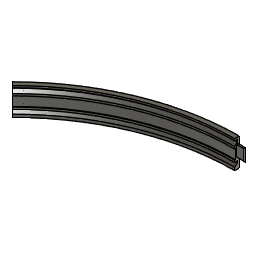
Model_Segment (Autodesk Fusion 360 design; units mm, degrees)
Autodesk Fusion 360 part; units mm, degrees
sketch "Sketch1" plane through (0, 0, 0) normal (0, 0, 1) x (1, 0, 0)
  circle A0 centre (0, 0) radius 246.5
  circle A1 centre (0, 0) radius 241.5
  line L0 (0, 350) -> (0, -350)
  line L1 (-247.4874, 247.4874) -> (247.4874, -247.4874)
  line L2 (-350, 0) -> (350, 0)
  line L3 (-247.4874, -247.4874) -> (247.4874, 247.4874)
  line L4 (0, 350) -> (0, -350)
  circle A2 centre (0, 0) radius 245
  dimension "d2" = 5
  dimension "d3" = 350
  dimension "d4" = 350
  dimension "d5" = 45
  dimension "d6" = 45
  dimension "d7" = 45
  dimension "d8" = 45
  dimension "d50" = 483
  dimension "d64" = 490
  constraint coincident A0.centre A1.centre
  constraint concentric A0 A1
  constraint vertical L0
  constraint vertical L4
  constraint concentric A0 A2
  measures "d2" distance of A0 A1
  measures "d3" distance of A0.centre L0.start
  measures "d4" distance of A0.centre L0.end
  measures "d5" angle of L0 L1
  measures "d6" angle of L1 L2
  measures "d7" angle of L2 L3
  measures "d8" angle of L3 L4
  measures "d50" diameter of A1
  measures "d64" diameter of A2
extrude "Extrude1" add sketch "Sketch1" along normal blind 30 contours A0 L0 L1 L4 A2 | A1 L0 L1 L4 A2 picked at (-21.3845, 244.5984) picked at (-130.7989, 205.231)
sketch "Sketch2" plane through (0, 0, 0) normal (1, 0, 0) x (0, 1, 0)
  line L0 (241.5, 0) -> (246.5, 0)
  line L1 (246.5, 0) -> (246.5, 30)
  line L2 (246.5, 30) -> (241.5, 30)
  line L3 (241.5, 30) -> (241.5, 0)
  line L4 (241.5, 28) -> (244.5, 28)
  line L5 (244.5, 28) -> (244.5, 25.5)
  line L6 (244.5, 6.1) -> (244.5, 7.6)
  line L7 (241.5, 20.3) -> (242.3, 20.3)
  line L8 (242.3, 20.3) -> (242.3, 9.8)
  line L9 (242.3, 9.8) -> (241.5, 9.8)
  line L10 (241.5, 9.8) -> (241.5, 20.3)
  line L11 (244.5, 6.1) -> (267.2426, 6.1) construction
  line L12 (244.5, 25.5) -> (241.5, 22.5)
  line L13 (244.5, 25.5) -> (267.2426, 25.5) construction
  line L14 (241.5, 28) -> (241.5, 22.5)
  line L15 (244.5, 7.6) -> (241.5, 7.6)
  line L16 (241.5, 7.6) -> (241.5, 3.1)
  line L17 (244.5, 6.1) -> (241.5, 3.1)
  dimension "d11" = 2
  dimension "d12" = 2
  dimension "d13" = 2.5
  dimension "d15" = 2
  dimension "d16" = 1.5
  dimension "d17" = 10.5
  dimension "d18" = 0.8
  dimension "d25" = 2.2
  dimension "d66" = 45
  dimension "d68" = 2.2
  dimension "d69" = 45
  constraint horizontal L4
  constraint vertical L5
  constraint coincident L3 L4.start
  constraint vertical L6
  constraint horizontal L7
  constraint vertical L8
  constraint horizontal L9
  constraint vertical L10
  constraint coincident L3 L7.start
  constraint horizontal L11
  constraint horizontal L13
  constraint coincident L3 L12.end
  constraint coincident L3 L15.end
  constraint perpendicular L3 L15
  constraint coincident L3 L16.end
  measures "d11" distance of L2 L4
  measures "d12" distance of L1 L5
  measures "d13" distance of L4.end L5.end
  measures "d15" distance of L1 L6
  measures "d16" distance of L6.start L6.end
  measures "d17" distance of L7.end L8.end
  measures "d18" distance of L8 L10
  measures "d25" distance of L7.start L12.end
  measures "d66" angle of L12 L14
  measures "d68" distance of L9.end L15.end
  measures "d69" angle of L16 L17
revolve "Revolve1" cut sketch "Sketch2" angle 360 about axis through (0, 0, 1.75) along (0, 0, 1) contours L3 L6 L15 L16 L17 | L3 L7 L8 L9 L10 | L3 L4 L5 L12 L14
sketch "Sketch3" plane through (0, 0, 0) normal (1, 0, 0) x (0, 1, 0)
  line L0 (244.5, 7.6) -> (244.5, 6.1)
  line L1 (241.5, 3.1) -> (241.5, 0)
  line L2 (241.5, 0) -> (246.5, 0)
  line L3 (246.5, 0) -> (246.5, 30)
  line L4 (246.5, 30) -> (241.5, 30)
  line L5 (241.5, 30) -> (241.5, 28)
  line L6 (241.5, 28) -> (244.5, 28)
  line L7 (244.5, 28) -> (244.5, 25.5)
  line L8 (244.5, 25.5) -> (241.5, 22.5)
  line L9 (241.5, 22.5) -> (241.5, 20.3)
  line L10 (241.5, 20.3) -> (242.3, 20.3)
  line L11 (242.3, 20.3) -> (242.3, 9.8)
  line L12 (242.3, 9.8) -> (241.5, 9.8)
  line L13 (245.2, 23.75) -> (243.4, 23.75)
  line L14 (245.2, 23.75) -> (245.2, 10.15)
  line L15 (245.2, 10.15) -> (243.4, 11.95)
  line L16 (245.2, 10.15) -> (249.7456, 10.15) construction
  line L17 (243.4, 23.75) -> (243.4, 11.95)
  line L18 (245.3, 23.85) -> (245.3, 9.85)
  line L19 (245.3, 9.85) -> (243.3, 11.85)
  line L20 (243.3, 11.85) -> (243.3, 23.85)
  line L21 (245.3, 23.85) -> (243.3, 23.85)
  line L22 (241.5, 7.6) -> (244.5, 7.6)
  line L23 (244.5, 6.1) -> (241.5, 3.1)
  line L24 (241.5, 9.8) -> (241.5, 7.6)
  dimension "d30" = 6.25
  dimension "d46" = 1.8
  dimension "d47" = 1.3
  dimension "d56" = 11.8
  dimension "d57" = 6.15
  dimension "d58" = 1.2
  dimension "d59" = 1.8
  dimension "d61" = 11.85
  dimension "d62" = 45
  dimension "d63" = 135
  constraint horizontal L13
  constraint perpendicular L13 L14
  constraint horizontal L16
  constraint perpendicular L13 L17
  constraint perpendicular L16 L18
  constraint perpendicular L20 L21
  measures "d30" distance of L4 L13
  measures "d46" distance of L14 L17
  measures "d47" distance of L3 L14
  measures "d56" distance of L13.end L15.end
  measures "d57" distance of L4 L21
  measures "d58" distance of L3 L18
  measures "d59" distance of L9 L20
  measures "d61" distance of L2 L19.end
  measures "d62" angle of L14 L15
  measures "d63" angle of L18 L19
revolve "Revolve2" add sketch "Sketch3" angle 1.9 about axis through (0, 0, 1.75) along (0, 0, -1) contours L13 L14 L15 L17
sketch "Sketch4" plane through (0, 0, 0) normal (-0.707107, -0.707107, 0) x (0.707107, -0.707107, 0)
  line L0 (-241.5, 7.6) -> (-241.5, 9.8)
  line L1 (-241.5, 9.8) -> (-242.3, 9.8)
  line L2 (-242.3, 9.8) -> (-242.3, 20.3)
  line L3 (-242.3, 20.3) -> (-241.5, 20.3)
  line L4 (-241.5, 20.3) -> (-241.5, 22.5)
  line L5 (-241.5, 22.5) -> (-244.5, 25.5)
  line L6 (-244.5, 25.5) -> (-244.5, 28)
  line L7 (-244.5, 28) -> (-241.5, 28)
  line L8 (-241.5, 28) -> (-241.5, 30)
  line L9 (-241.5, 30) -> (-246.5, 30)
  line L10 (-246.5, 30) -> (-246.5, 0)
  line L11 (-246.5, 0) -> (-241.5, 0)
  line L12 (-241.5, 0) -> (-241.5, 3.1)
  line L13 (-244.5, 6.1) -> (-244.5, 7.6)
  line L14 (-245.3, 23.85) -> (-243.3, 23.85)
  line L15 (-245.3, 9.85) -> (-245.3, 23.85)
  line L16 (-245.3, 9.85) -> (-243.3, 11.85)
  line L17 (-245.3, 9.85) -> (-242.4716, 9.85) construction
  line L18 (-243.3, 23.85) -> (-243.3, 11.85)
  line L19 (-244.5, 7.6) -> (-241.5, 7.6)
  line L20 (-241.5, 3.1) -> (-244.5, 6.1)
  dimension "d38" = 14
  dimension "d39" = 2
  dimension "d40" = 1.2
  dimension "d42" = 6.15
  dimension "d55" = 12
  dimension "d70" = 45
  constraint horizontal L14
  constraint vertical L15
  constraint horizontal L17
  constraint perpendicular L14 L18
  measures "d38" distance of L14.start L15.start
  measures "d39" distance of L14.start L14.end
  measures "d40" distance of L10 L15
  measures "d42" distance of L9 L14
  measures "d55" distance of L14.end L16.end
  measures "d70" angle of L15 L16
revolve "Revolve3" cut sketch "Sketch4" angle 2 about axis through (0, 0, 1.75) along (0, 0, -1) contours L14 L15 L16 L18
